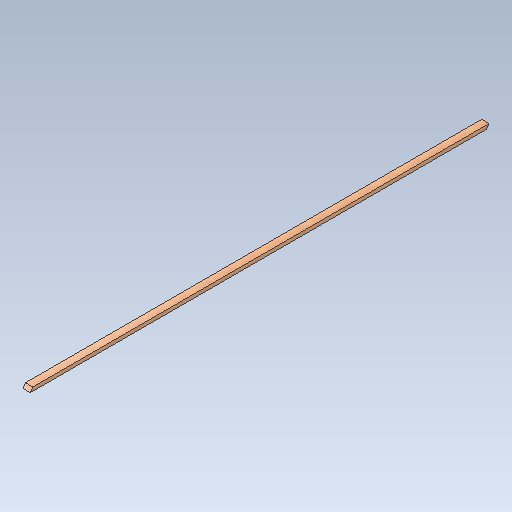
# Autodesk Inventor part: træhåndfang
Saved by Autodesk Inventor 2020.1 (Build 241239000, 239)
## iProperties
Created: 2019-09-28
Part Number: træhåndfang
Material: Wood (Birch)
Document SubType Name: Modeling
Designer: loppen
Density: 0.55 g/cm^3
Appearance: Birch - Natural Polished
Mass: 11829.5 g
Surface Area: 12525.9 cm^2
Volume: 21508.1 cm^3
Author: loppen
Autodesk Inventor part; units mm, degrees
ref_plane "YZ Plane" through (0, 0, 0) normal (1, 0, 0) x (0, 1, 0)
ref_plane "XZ Plane" through (0, 0, 0) normal (0, 1, 0) x (-1, 0, 0)
ref_plane "XY Plane" through (0, 0, 0) normal (0, 0, 1) x (1, 0, 0)
sketch "Sketch1" plane through (0, 0, 0) normal (0, 0, 1) x (1, 0, 0)
  line L0 (-56, 0) -> (56, 0) projected
  line L1 (40, -20) -> (40, 20)
  line L2 (40, 20) -> (-40, 20)
  line L3 (-40, 20) -> (-40, -20)
  line L4 (-40, -20) -> (40, -20)
  point P0 (0, 0)
  dimension "d8" = 80
  dimension "d9" = 40
  dimension "d11" = 40
  constraints: 8 end point, 1 horizontal, 1 parallel, 1 perpendicular, 1 other
  measures "d8" distance of L1.end L2.end
  measures "d9" distance of L1.start L1.end
  measures "d11" distance from line of point (0, 0) L3
extrude "brædt" add sketch "Sketch1" along normal mid plane 5000
sketch "Sketch2" plane through (40, -20, -2500) normal (0, -1, 0) x (1, 0, 0)
  line L0 (0, 5000) -> (0, 0) projected
  line L1 (-80, 5000) -> (0, 5000) projected
  line L2 (-80, 0) -> (-80, 5000) projected
  line L3 (0, 0) -> (-80, 0) projected
  line L4 (-40, -1000) -> (-40, 6000) projected
  line L5 (-12.25, 69.175) -> (-67.75, 69.175)
  line L6 (-70.75, 72.175) -> (-70.75, 4910.726)
  line L7 (-67.75, 4913.726) -> (-12.25, 4913.726)
  line L8 (-9.25, 4910.726) -> (-9.25, 72.175)
  arc A0 (-70.75, 72.175) -> (-67.75, 69.175) centre (-67.75, 72.175) ccw
  arc A1 (-12.25, 69.175) -> (-9.25, 72.175) centre (-12.25, 72.175) ccw
  arc A2 (-67.75, 4913.726) -> (-70.75, 4910.726) centre (-67.75, 4910.726) ccw
  arc A3 (-9.25, 4910.726) -> (-12.25, 4913.726) centre (-12.25, 4910.726) ccw
  point P0 (-40, 2500)
  dimension "d12" = 61.5
  dimension "d13" = 4844.551
  dimension "d14" = 3
  dimension "d29" = 69.175
  constraints: 8 end point, 8 point on circle, 8 tangent, 4 centre point, 3 equal radius, 2 parallel, 1 horizontal, 1 perpendicular, 1 other
  measures "d12" distance between parallel lines of L8 L6
  measures "d13" distance between parallel lines of L7 L5
  measures "d14" radius of A0
  measures "d29" distance between parallel lines of L3 L5
extrude "spor til stål-håndfang" cut sketch "Sketch2" against normal blind 5 contours L7 A3 L8 A1 L5 L4 | L4 L5 A0 L6 A2 L7
sketch "Sketch3" plane through (40, -15, -2500) normal (0, -1, 0) x (1, 0, 0)
  line L0 (-70.75, 72.175) -> (-70.75, 4910.726) projected
  arc A0 (-70.75, 72.175) -> (-67.75, 69.175) centre (-67.75, 72.175) ccw projected
  line L1 (-12.25, 69.175) -> (-67.75, 69.175) projected
  arc A1 (-12.25, 69.175) -> (-9.25, 72.175) centre (-12.25, 72.175) ccw projected
  line L2 (-9.25, 4910.726) -> (-9.25, 72.175) projected
  arc A2 (-9.25, 4910.726) -> (-12.25, 4913.726) centre (-12.25, 4910.726) ccw projected
  line L3 (-67.75, 4913.726) -> (-12.25, 4913.726) projected
  arc A3 (-67.75, 4913.726) -> (-70.75, 4910.726) centre (-67.75, 4910.726) ccw projected
  line L4 (-40, 4906.726) -> (-40, 76.175) construction
  line L5 (-46, 4906.726) -> (-46, 76.175)
  line L6 (-34, 76.175) -> (-34, 4906.726)
  arc A4 (-34, 4906.726) -> (-46, 4906.726) centre (-40, 4906.726) ccw
  arc A5 (-46, 76.175) -> (-34, 76.175) centre (-40, 76.175) ccw
  line L7 (-40, -1000) -> (-40, 6000) projected
  point P0 (-40, 2500)
  point P1 (-40, 2491.4505)
  dimension "d19" = 12
  dimension "d22" = 1
  dimension "d23" = 1
  constraints: 8 end point, 4 point on circle, 4 tangent, 2 centre point, 1 collinear, 1 midpoint, 1 parallel, 1 vertical
  measures "d19" diameter of A5
  measures "d22" distance edge to line of A5 L1
  measures "d23" distance edge to line of A4 L3
extrude "spor til LED og liste" cut sketch "Sketch3" against normal blind 12 contours L7 A4 L6 A5 | A5 L5 A4 L7
sketch "Sketch4" plane through (40, -3, -2500) normal (0, -1, 0) x (1, 0, 0)
  line L0 (-46, 76.175) -> (-46, 4906.726) projected
  arc A0 (-46, 76.175) -> (-34, 76.175) centre (-40, 76.175) ccw projected
  line L1 (-34, 4906.726) -> (-34, 76.175) projected
  arc A1 (-34, 4906.726) -> (-46, 4906.726) centre (-40, 4906.726) ccw projected
  line L2 (-40, -1000) -> (-40, 6000) projected
  line L3 (-40, 4907.726) -> (-40, 75.175) construction
  line L4 (-45, 4907.726) -> (-45, 75.175)
  line L5 (-35, 75.175) -> (-35, 4907.726)
  arc A2 (-35, 4907.726) -> (-45, 4907.726) centre (-40, 4907.726) ccw
  arc A3 (-45, 75.175) -> (-35, 75.175) centre (-40, 75.175) ccw
  point P0 (-40, 2500)
  point P1 (-40, 2491.4505)
  dimension "d24" = 10
  dimension "d25" = 0
  dimension "d26" = 0
  constraints: 8 end point, 4 point on circle, 4 tangent, 2 centre point, 2 point on line, 1 midpoint, 1 parallel
  measures "d24" diameter of A3
  measures "d25" horizontal distance between centres of A0 A3
  measures "d26" horizontal distance between centres of A1 A2
extrude "spor til ledninger" cut sketch "Sketch4" against normal blind 7 contours A3 L4 A2 L2 | L2 A2 L5 A3
sketch "Sketch5" plane through (40, 20, 2500) normal (1, 0, 0) x (0, 0, -1)
  line L0 (0, 0) -> (5000, 0) projected
  line L1 (0, -40) -> (0, 0) projected
  line L2 (0, -40) -> (5000, -40) projected
  line L3 (5000, 0) -> (5000, -40) projected
  line L4 (5000, 0) -> (5000, -40) projected
  line L5 (5000, 0) -> (4972.7139, -40)
  line L6 (0, -40) -> (5000, -40) projected
  point P0 (2500, -20)
  dimension "d30" = 34.3
  constraints: 2 end point, 1 point on line
  measures "d30" angle of L3 L5
extrude "endeafskær top" cut sketch "Sketch5" against normal through all contours L3 L2 L5
sketch "Sketch6" plane through (40, 20, 2500) normal (1, 0, 0) x (0, 0, -1)
  line L0 (4972.7139, -40) -> (5000, 0) projected
  line L1 (0, 0) -> (5000, 0) projected
  line L2 (0, -40) -> (0, 0) projected
  line L3 (0, -40) -> (4972.7139, -40) projected
  line L4 (0, -40) -> (0, 0) projected
  line L5 (0, -40) -> (27.2861, 0)
  point P0 (2500, -20)
  dimension "d33" = 34.3
  constraints: 2 end point, 1 point on line
  measures "d33" angle of L2 L5
extrude "endeafskær bund" cut sketch "Sketch6" against normal through all contours L2 L1 L5
fillet "Fillet2" [suppressed]
fillet "Fillet3" [suppressed]
fillet "Fillet4" [suppressed]
fillet "Fillet5" [suppressed]
sketch "Sketch7" plane through (40, -15, -2500) normal (0, -1, 0) x (1, 0, 0)
  ellipse E0 centre (-40, 566.2041) end of major axis (-40, 591.0196) minor radius 20.5 projected
  ellipse E1 centre (-40, 1776.9092) end of major axis (-40, 1801.7247) minor radius 20.5 projected
  ellipse E2 centre (-40, 2987.8572) end of major axis (-40, 3012.6727) minor radius 20.5 projected
  line L0 (-93.9939, 549.6501) -> (45.3161, 549.6501) construction
  line L1 (-103.3896, 1760.3552) -> (51.928, 1760.3552) construction
  line L2 (-132.8398, 2971.3032) -> (53.2138, 2971.3032) construction
  line L3 (-45, 75.175) -> (-45, 4907.726) construction
  arc A0 (-45, 75.175) -> (-35, 75.175) centre (-40, 75.175) ccw construction
  line L4 (-35, 4907.726) -> (-35, 75.175) construction
  arc A1 (-35, 4907.726) -> (-45, 4907.726) centre (-40, 4907.726) ccw construction
  circle A2 centre (-45, 549.6501) radius 6
  circle A3 centre (-35, 549.6501) radius 6
  circle A4 centre (-35, 1760.3552) radius 6
  circle A5 centre (-45, 1760.3552) radius 6
  circle A6 centre (-45, 2971.3032) radius 6
  circle A7 centre (-35, 2971.3032) radius 6
  point P0 (-40, 2500)
  dimension "d38" = 12
  dimension "d39" = 12
  dimension "d40" = 12
  dimension "d41" = 12
  dimension "d42" = 12
  dimension "d43" = 12
  constraints: 12 point on line, 6 centre point, 6 end point, 3 horizontal, 3 other
  measures "d38" diameter of A2
  measures "d39" diameter of A3
  measures "d40" diameter of A4
  measures "d41" diameter of A5
  measures "d42" diameter of A6
  measures "d43" diameter of A7
extrude "pilothuller" cut sketch "Sketch7" against normal up to surface (19 mm away) contours A2 A3 | A2 A3 | A3 A2 | A4 A5 | A5 A4 | A4 A5 | A6 A7 | A6 A7 | A7 A6
sketch "Sketch8" plane through (40, -15, -2500) normal (0, -1, 0) x (1, 0, 0)
  line L0 (-70.75, 72.175) -> (-70.75, 4910.726) projected
  arc A0 (-70.75, 72.175) -> (-67.75, 69.175) centre (-67.75, 72.175) ccw projected
  line L1 (-12.25, 69.175) -> (-67.75, 69.175) projected
  arc A1 (-12.25, 69.175) -> (-9.25, 72.175) centre (-12.25, 72.175) ccw projected
  line L2 (-9.25, 4910.726) -> (-9.25, 72.175) projected
  arc A2 (-9.25, 4910.726) -> (-12.25, 4913.726) centre (-12.25, 4910.726) ccw projected
  line L3 (-67.75, 4913.726) -> (-12.25, 4913.726) projected
  arc A3 (-67.75, 4913.726) -> (-70.75, 4910.726) centre (-67.75, 4910.726) ccw projected
  arc A4 (-34, 543.734) -> (-34, 555.5662) centre (-35, 549.6501) ccw projected
  line L4 (-34, 543.734) -> (-34, 76.175) projected
  arc A5 (-46, 76.175) -> (-34, 76.175) centre (-40, 76.175) ccw projected
  line L5 (-46, 76.175) -> (-46, 543.734) projected
  arc A6 (-46, 555.5662) -> (-46, 543.734) centre (-45, 549.6501) ccw projected
  line L6 (-46, 555.5662) -> (-46, 1754.4392) projected
  arc A7 (-46, 1766.2713) -> (-46, 1754.4392) centre (-45, 1760.3552) ccw projected
  line L7 (-46, 1766.2713) -> (-46, 2965.3872) projected
  arc A8 (-46, 2977.2193) -> (-46, 2965.3872) centre (-45, 2971.3032) ccw projected
  line L8 (-46, 2977.2193) -> (-46, 4906.726) projected
  arc A9 (-34, 4906.726) -> (-46, 4906.726) centre (-40, 4906.726) ccw projected
  line L9 (-34, 4906.726) -> (-34, 2977.2193) projected
  arc A10 (-34, 2965.3872) -> (-34, 2977.2193) centre (-35, 2971.3032) ccw projected
  line L10 (-34, 2965.3872) -> (-34, 1766.2713) projected
  arc A11 (-34, 1754.4392) -> (-34, 1766.2713) centre (-35, 1760.3552) ccw projected
  line L11 (-34, 1754.4392) -> (-34, 555.5662) projected
  line L12 (-49, 4913.726) -> (-31, 4913.726)
  line L13 (-28, 4910.726) -> (-28, 72.175)
  line L14 (-31, 69.175) -> (-49, 69.175)
  line L15 (-52, 72.175) -> (-52, 4910.726)
  line L16 (-40, -1000) -> (-40, 6000) construction
  arc A12 (-28, 4910.726) -> (-31, 4913.726) centre (-31, 4910.726) ccw
  arc A13 (-49, 4913.726) -> (-52, 4910.726) centre (-49, 4910.726) ccw
  arc A14 (-31, 69.175) -> (-28, 72.175) centre (-31, 72.175) ccw
  arc A15 (-52, 72.175) -> (-49, 69.175) centre (-49, 72.175) ccw
  point P0 (-40, 2500)
  point P1 (-52, 4913.726)
  point P2 (-28, 4913.726)
  dimension "d46" = 24
  dimension "d47" = 3
  dimension "d52" = 0
  dimension "d53" = 0
  constraints: 8 end point, 8 point on circle, 8 tangent, 4 centre point, 4 point on line, 3 equal radius, 2 parallel, 1 horizontal, 1 perpendicular, 1 other
  measures "d46" distance of point (-52, 4913.726) point (-28, 4913.726)
  measures "d47" radius of A12
  measures "d52" distance between parallel lines of L1 L14
  measures "d53" distance between parallel lines of L3 L12
extrude "spor til acryl" cut sketch "Sketch8" against normal blind 2 contours A15 L15 A13 L3 A12 L13 A14 L1 | L4 A5 L5 A6 L6 A7 L7 A8 L8 A9 L9 A10 L10 A11 L11 A4
equation "\"d11\" = 0.5 * d8"
equation "\"d30\" = trappevinkel"
equation "\"d33\" = trappevinkel"
equation "\"d39\" = d38"
equation "\"d40\" = d38"
equation "\"d41\" = d38"
equation "\"d42\" = d38"
equation "\"d43\" = d38"
equation "\"pladetykkelse\" = 3"
equation "\"trappevinkel\" = 34.3deg"
equation "\"trappestifter_dia\" = 25"
equation "\"trappestifter_huldia\" = 25.8"
equation "\"trappestifter_skraa_huldia\" = 26.6"
equation "\"trappestifter_laengde\" = 228"
equation "\"perforeringsbredde\" = 6"
equation "\"perforeringshullaengde\" = 62.8"
equation "\"perforeringshullaengde_top\" = 61"
equation "\"perforeringshullaengde_bund\" = 61.6"
equation "\"perforeringsoffset\" = 8"
equation "\"perforeringsoffset_top\" = 8"
equation "\"perforeringsoffset_bund\" = 8"
equation "\"laskehul_dia\" = 13"
equation "\"balusterhul_udvidelse\" = 1"
equation "\"trinbredde\" = 1884"
body "Solid1"
